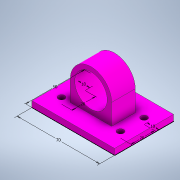
# Autodesk Inventor part: base_motor
Saved by Autodesk Inventor 2022 (Build 260153000, 153)
## iProperties
Created: 2022-02-18
Part Number: base_motor
Material: Generic
Document SubType Name: Modeling
Designer: Home
Density: 1 g/cm^3
Appearance: Default
Author: Home
Autodesk Inventor part; units mm, degrees
ref_plane "YZ Plane" through (0, 0, 0) normal (1, 0, 0) x (0, 1, 0)
ref_plane "XZ Plane" through (0, 0, 0) normal (0, 1, 0) x (-1, 0, 0)
ref_plane "XY Plane" through (0, 0, 0) normal (0, 0, 1) x (1, 0, 0)
sketch "Sketch1" plane through (0, 0, 0) normal (0, 1, 0) x (-1, 0, 0)
  line L0 (-35, -25) -> (35, -25)
  line L1 (35, -25) -> (35, 25)
  line L2 (35, 25) -> (-35, 25)
  line L3 (-35, 25) -> (-35, -25)
  line L4 (-35, -25) -> (35, 25) construction
  line L5 (35, -25) -> (-35, 25) construction
  line L6 (25, -10) -> (25, 10)
  line L7 (-25, -10) -> (-25, 10)
  point P0 (0, 0)
  point P1 (25, 0)
  point P2 (0, 0)
  point P3 (-25, 0)
  dimension "d0" = 70
  dimension "d1" = 50
  dimension "d17" = 20
  dimension "d18" = 20
  dimension "d19" = 10
  dimension "d20" = 10
  constraints: 16 end point, 5 midpoint, 2 horizontal alignment, 2 parallel, 2 vertical, 1 horizontal, 1 perpendicular
  measures "d0" distance of L2.end L1.end
  measures "d1" distance of L1.end L0.end
  measures "d17" distance of L6.start L6.end
  measures "d18" distance of L7.start L7.end
  measures "d19" distance from line of L1 L6.start
  measures "d20" distance from line of L3 L7.start
extrude "Extrusion1" add sketch "Sketch1" along normal blind 5
sketch "Sketch3" plane through (0, 0, 0) normal (0, 0, 1) x (1, 0, 0)
  circle A0 centre (0, 22.5) radius 17.5
  line L0 (-35, 5) -> (35, 5) projected
  circle A1 centre (0, 22.5) radius 13.75
  line L1 (17.5, 22.5) -> (17.5, 5)
  line L2 (-17.5, 22.5) -> (-17.5, 5)
  point P0 (0, 0)
  point P1 (0, 5)
  point P2 (0, 5)
  dimension "d13" = 35
  dimension "d14" = 27.5
  constraints: 4 end point, 3 point on circle, 2 centre point, 2 midpoint, 2 point on line, 1 coincident, 1 horizontal alignment, 1 perpendicular, 1 tangent, 1 vertical, 1 vertical alignment
  measures "d13" diameter of A0
  measures "d14" diameter of A1
extrude "Extrusion2" add sketch "Sketch3" along normal mid plane 20
hole "Hole2" at (-25, 0, -10) at (-25, 0, 10) at (25, 0, -10) at (25, 0, 10) direction (0, 1, 0) diameter 5.4 end through all
body "Solid1"
